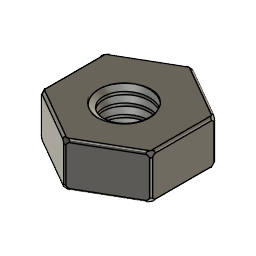
M2.5 Hex Nut (Autodesk Fusion 360 design; units mm, degrees)
Autodesk Fusion 360 part; units mm, degrees
sketch "Sketch1" plane through (0, 0, 0) normal (0, 0, 1) x (1, 0, 0)
  line L0 (2.5, 1.4434) -> (0, 2.8868)
  line L1 (0, 2.8868) -> (-2.5, 1.4434)
  line L2 (-2.5, 1.4434) -> (-2.5, -1.4434)
  line L3 (-2.5, -1.4434) -> (0, -2.8868)
  line L4 (0, -2.8868) -> (2.5, -1.4434)
  line L5 (2.5, -1.4434) -> (2.5, 1.4434)
  circle A0 centre (0, 0) radius 1.25
  dimension "d22" = 2.5
  constraint coincident A0.centre origin
  measures "d22" diameter of A0
extrude "Extrude1" add sketch "Sketch1" along normal blind 2 contours L0 L1 L2 L3 L4 L5 | A0
sketch "Sketch2" plane through (2.5, 0, 0) normal (1, 0, 0) x (0, 1, 0)
  line L0 (-1.4434, 0) -> (1.4434, 0)
  line L1 (1.4434, 0) -> (1.4434, 2)
  line L2 (1.4434, 2) -> (-1.4434, 2)
  line L3 (-1.4434, 2) -> (-1.4434, 0)
  line L4 (-1.4434, 2) -> (-1.4434, 1.75)
  line L5 (-1.4434, 0) -> (-1.4434, 0.25)
  dimension "d5" = 0.25
  dimension "d6" = 0.25
  constraint coincident L2.end L3.start
  constraint perpendicular L2 L4
  constraint coincident L0.start L3.end
  constraint perpendicular L0 L5
  measures "d5" distance of L2.end L4.end
  measures "d6" distance of L0.start L5.end
sketch "Sketch3" plane through (0, 0, 2) normal (0, 0, 1) x (-1, 0, 0)
  line L0 (-2.5, 1.4434) -> (-2.5, -1.4434)
  line L1 (-2.5, -1.4434) -> (0, -2.8868)
  line L2 (0, -2.8868) -> (2.5, -1.4434)
  line L3 (2.5, -1.4434) -> (2.5, 1.4434)
  line L4 (2.5, 1.4434) -> (0, 2.8868)
  line L5 (0, 2.8868) -> (-2.5, 1.4434)
  line L6 (-2.5, 1.4434) -> (-2.5, 1.1934)
  line L7 (-2.5, 1.4434) -> (-2.2835, 1.5684)
  dimension "d7" = 0.25
  dimension "d8" = 0.25
  constraint coincident L0.start L5.end
  constraint parallel L0 L6
  constraint parallel L5 L7
  measures "d7" distance of L0.start L6.end
  measures "d8" distance of L0.start L7.end
sketch "Sketch4" plane through (0, 0, 0) normal (0, 0, -1) x (1, 0, 0)
  line L0 (2.5, -1.4434) -> (2.5, 1.4434)
  line L1 (2.5, 1.4434) -> (0, 2.8868)
  line L2 (0, 2.8868) -> (-2.5, 1.4434)
  line L3 (-2.5, 1.4434) -> (-2.5, -1.4434)
  line L4 (-2.5, -1.4434) -> (0, -2.8868)
  line L5 (0, -2.8868) -> (2.5, -1.4434)
  line L6 (2.5, 1.4434) -> (2.2835, 1.5684)
  line L7 (2.5, 1.4434) -> (2.5, 1.1934)
  dimension "d9" = 0.25
  dimension "d10" = 0.25
  constraint coincident L0.end L1.start
  constraint parallel L1 L6
  constraint parallel L0 L7
  measures "d9" distance of L0.end L6.end
  measures "d10" distance of L0.end L7.end
ref_plane "WorkPlane1" through (2.5, -1.4434, 0.25) normal (-0.774597, 0.447214, 0.447214) x (0.5, 0, 0.866025)
ref_plane "WorkPlane2" through (2.2835, -1.5684, 2) normal (-0.774597, 0.447214, -0.447214) x (-0.5, 0, 0.866025)
sketch "Sketch5" plane through (2.6062, -1.5047, 1.5047) normal (-0.774597, 0.447214, -0.447214) x (-0.5, 0, 0.866025)
  line L0 (0.65, 0.35) -> (0.25, 0.35)
  line L1 (0.25, 0.35) -> (0.25, -0.1)
  line L2 (0.25, -0.1) -> (0.65, -0.1)
  line L3 (0.65, -0.1) -> (0.65, 0.35)
  constraint horizontal L0
  constraint vertical L1
  constraint horizontal L2
  constraint vertical L3
extrude "Extrude2" cut sketch "Sketch5" against normal blind 5
sketch "Sketch6" plane through (1.9134, -1.1047, -1.1047) normal (-0.774597, 0.447214, 0.447214) x (0.5, 0, 0.866025)
  line L0 (1.5, -0.05) -> (1.1, -0.05)
  line L1 (1.1, -0.05) -> (1.1, -0.55)
  line L2 (1.1, -0.55) -> (1.5, -0.55)
  line L3 (1.5, -0.55) -> (1.5, -0.05)
  constraint horizontal L0
  constraint vertical L1
  constraint horizontal L2
  constraint vertical L3
extrude "Extrude3" cut sketch "Sketch6" against normal blind 5
pattern_circular "C-Pattern1" count 6 over 360 about axis through (0, 0, 1.75) along (0, 0, 1) of "Extrude2", "Extrude3"
extrude "Extrude4" cut sketch "Sketch1" along normal blind 2 contours A0
fillet "Fillet1" radius 0.1 18 edges at (-2.5, 1.4434, 1) (-2.5, -1.4434, 1) (0, -2.8868, 1) (2.5, -1.4434, 1) (2.5, 1.4434, 1) (0, 2.8868, 1) (1.25, 2.1651, 2) (-1.25, 2.1651, 2) (2.5, 0, 2) (1.25, -2.1651, 2) (-1.25, -2.1651, 2) (-2.5, 0, 2) (-1.25, -2.1651, 0) (1.25, -2.1651, 0) (2.5, 0, 0) (1.25, 2.1651, 0) (-1.25, 2.1651, 0) (-2.5, 0, 0)
thread "Thread1" "ISO Metric profile 2.5 M2.5x0.45 M2.5x0.45 6H" major diameter 2.58 minor diameter 2.0755 pitch 0.45 angle 60 modelled right hand crest width 0.1211 on face at (1.2484, -0.0623, 1.3333) crest through (1.0377, 0, 0.1125)
